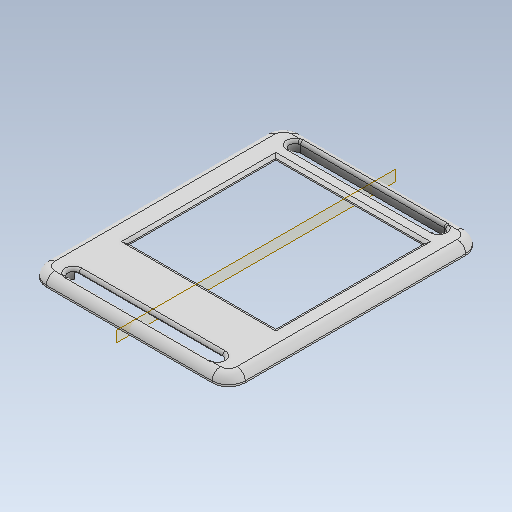
# Autodesk Inventor part: Top
Saved by Autodesk Inventor 2020.1 (Build 241239000, 239)
## iProperties
Created: 2021-08-24
Part Number: Top
Material: Generic
Document SubType Name: Modeling
Designer: nigel
Density: 1 g/cm^3
Appearance: Default
Author: nigel
Autodesk Inventor part; units mm, degrees
ref_plane "XZ Plane" through (0, 0, 0) normal (0, 1, 0) x (-1, 0, 0)
ref_plane "XY Plane" through (0, 0, 0) normal (0, 0, 1) x (1, 0, 0)
sketch "Sketch1" plane through (0, 0, 0) normal (0, 1, 0) x (-1, 0, 0)
  line L0 (18, 22.95) -> (-18, 22.95)
  line L1 (-18, 22.95) -> (-18, -22.95)
  line L2 (-18, -22.95) -> (18, -22.95)
  line L3 (18, -22.95) -> (18, 22.95)
  line L4 (18, 22.95) -> (-18, -22.95) construction
  line L5 (-18, 22.95) -> (18, -22.95) construction
  line L6 (14, -19.05) -> (-14, -19.05)
  line L7 (-14, -19.05) -> (-14, -21.05)
  line L8 (-14, -21.05) -> (14, -21.05)
  line L9 (14, -21.05) -> (14, -19.05)
  line L10 (14, -19.05) -> (-14, -21.05) construction
  line L11 (-14, -19.05) -> (14, -21.05) construction
  line L12 (14, 21.05) -> (-14, 21.05)
  line L13 (-14, 21.05) -> (-14, 19.05)
  line L14 (-14, 19.05) -> (14, 19.05)
  line L15 (14, 19.05) -> (14, 21.05)
  line L16 (14, 21.05) -> (-14, 19.05) construction
  line L17 (-14, 21.05) -> (14, 19.05) construction
  line L18 (15.6, 19.25) -> (-16.5, 19.25)
  line L19 (-16.5, 19.25) -> (-16.5, -19.25)
  line L20 (-16.5, -19.25) -> (15.6, -19.25)
  line L21 (15.6, -19.25) -> (15.6, 19.25)
  line L22 (12.95, 10.25) -> (-13.85, 10.25)
  line L23 (-13.85, 10.25) -> (-13.85, -16.55)
  line L24 (-13.85, -16.55) -> (12.95, -16.55)
  line L25 (12.95, -16.55) -> (12.95, 10.25)
  point P0 (0, 0)
  point P1 (0, -20.05)
  point P2 (0, 20.05)
  point P3 (0, 20.05)
  point P4 (0, 0)
  point P5 (0, 0)
  point P6 (0, -20.05)
  point P7 (-0.45, 10.25)
  point P8 (-0.45, -19.25)
  point P9 (-14, 19.25)
  point P10 (14, 19.25)
  point P11 (14, -19.25)
  point P12 (-14, -19.25)
  dimension "d0" = 45.9
  dimension "d1" = 1.9
  dimension "d2" = 2
  dimension "d3" = 2
  dimension "d4" = 1.9
  dimension "d5" = 28
  dimension "d6" = 36
  dimension "d7" = 32.1
  dimension "d8" = 38.5
  dimension "d10" = 2.4
  dimension "d11" = 26.8
  dimension "d12" = 26.8
  dimension "d13" = 2.5
  dimension "d21" = 0.2
  constraints: 52 end point, 12 midpoint, 10 parallel, 5 horizontal, 5 perpendicular, 3 vertical alignment, 1 point on line
  measures "d0" distance of L2.end L0.start
  measures "d1" distance between parallel lines of L0 L12
  measures "d2" distance of L14.end L12.start
  measures "d3" distance of L8.end L6.start
  measures "d4" distance between parallel lines of L2 L8
  measures "d5" distance of L7.end L8.end
  measures "d6" distance of L0.start L0.end
  measures "d7" distance of L18.start L18.end
  measures "d8" distance of L18.end L19.end
  measures "d10" distance between parallel lines of L3 L21
  measures "d11" distance of L24.end L22.start
  measures "d12" distance of L23.end L24.end
  measures "d13" distance between parallel lines of L24 L6
  measures "d21" distance between parallel lines of L20 L6
extrude "Extrusion1" add sketch "Sketch1" along normal blind 1.8 contours L3 L2 L1 L0 | L6 L7 L20 L19 L18 L13 L14 L15 L21 L9
extrude "Extrusion2" cut sketch "Sketch1" along normal blind 1.2 contours L6 L7 L20 L19 L18 L13 L14 L15 L21 L9
fillet "Fillet1" radius 3 4 edges at (18, 0.9, 22.95) (18, 0.9, -22.95) (-18, 0.9, -22.95) (-18, 0.9, 22.95)
fillet "Fillet1" radius 1 8 edges at (-14, 0.9, -21.05) (-14, 1.5, -19.05) (14, 0.9, -21.05) (14, 1.5, -19.05) (14, 0.9, 21.05) (14, 1.5, 19.05) (-14, 1.5, 19.05) (-14, 0.9, 21.05)
fillet "Fillet2" radius 1.5 8 edges at (-17.1213, 1.8, 22.0713) (0, 1.8, 22.95) (17.1213, 1.8, 22.0713) (18, 1.8, 0) (17.1213, 1.8, -22.0713) (0, 1.8, -22.95) (-17.1213, 1.8, -22.0713) (-18, 1.8, 0)
chamfer "Chamfer1" distance 0.6 angle 30 4 edges at (13.85, 1.8, -3.15) (0.45, 1.8, -16.55) (0.45, 1.8, 10.25) (-12.95, 1.8, -3.15) measured on face at (0.45, 1.8, 10.75) measured on face at (0.45, 1.8, -17.05) measured on face at (14.35, 1.8, -3.15) measured on face at (-13.45, 1.8, -3.15)
fillet "Fillet3" radius 0.5 16 edges at (-13.7071, 1.8, 19.3429) (-13.7071, 1.8, 20.7571) (-14, 1.8, 20.05) (0, 1.8, 19.05) (14, 1.8, 20.05) (13.7071, 1.8, 19.3429) (13.7071, 1.8, 20.7571) (0, 1.8, 21.05) (-13.7071, 1.8, -19.3429) (-14, 1.8, -20.05) (-13.7071, 1.8, -20.7571) (0, 1.8, -21.05) (13.7071, 1.8, -19.3429) (14, 1.8, -20.05) (13.7071, 1.8, -20.7571) (0, 1.8, -19.05)
equation "\"d3\" = d2"
equation "\"d4\" = d1"
equation "\"d12\" = d11"
body "Solid1"
